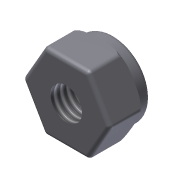
# Autodesk Inventor part: 10-32 regular lock nut
Saved by Autodesk Inventor 2013 (Build 170138000, 138)
## iProperties
Created: 2011-07-10
Part Number: 10-32 regular lock nut
Document SubType Name: Modeling
Designer: Dan Niemitalo
Density: 3.73276 g/cm^3
Material: Steel
Mass: 1.361 g
Surface Area: 3.79246 cm^2
Volume: 0.364609 cm^3
Author: Dan Niemitalo
Autodesk Inventor part; units mm, degrees
ref_plane "YZ Plane" through (0, 0, 0) normal (1, 0, 0) x (0, 1, 0)
ref_plane "XZ Plane" through (0, 0, 0) normal (0, 1, 0) x (-1, 0, 0)
ref_plane "XY Plane" through (0, 0, 0) normal (0, 0, 1) x (1, 0, 0)
sketch "Sketch1" plane through (0, 0, 0) normal (0, 0, 1) x (1, 0, 0)
  line L0 (-2.7496, 4.7625) -> (2.7496, 4.7625)
  line L1 (2.7496, 4.7625) -> (5.4993, 0)
  line L2 (5.4993, 0) -> (2.7496, -4.7625)
  line L3 (2.7496, -4.7625) -> (-2.7496, -4.7625)
  line L4 (-2.7496, -4.7625) -> (-5.4993, 0)
  line L5 (-5.4993, 0) -> (-2.7496, 4.7625)
  point P0 (0, 0)
  point P1 (0, 0)
  dimension "d0" = 9.525
  constraints: 12 end point, 1 coincident, 1 horizontal, 13 other
  measures "d0" distance between parallel lines of L3 L0
extrude "Extrusion1" add sketch "Sketch1" along normal blind 4.3656
sketch "Sketch3" plane through (0, 0, 4.3656) normal (0, 0, 1) x (1, 0, 0)
  circle A0 centre (0, 0) radius 4.572
  dimension "d3" = 9.144
  constraints: 1 centre point, 1 coincident
  measures "d3" diameter of A0
extrude "Extrusion2" add sketch "Sketch3" along normal blind 1.5875
sketch "Sketch8" plane through (0, 0, 5.9531) normal (0, 0, 1) x (1, 0, 0)
  circle A0 centre (0, 0) radius 1.9812 projected
  circle A1 centre (0, 0) radius 4.572 projected
  circle A2 centre (0, 0) radius 3.175
  dimension "d14" = 6.35
  constraints: 1 centre point, 1 coincident
  measures "d14" diameter of A2
extrude "Extrusion3" cut sketch "Sketch8" against normal blind 0.254 contours A2
sketch "Sketch9" plane through (0, 0, 0) normal (0, 0, -1) x (-1, 0, 0)
  point P0 (0, 0)
hole "Hole2" at (0, 0, 0) direction (0, 0, 1) diameter 3.9624 end through all thread size "10-32 UNF" class "2B" standard "ANSI Unified Screw Threads"
sketch "Sketch10" plane through (0, 0, 0) normal (0, 1, 0) x (-1, 0, 0)
  line L0 (-5.4993, 4.3656) -> (-2.7496, 4.3656) projected
  line L1 (-2.7496, 0) -> (-2.7496, 4.3656) projected
  line L2 (-5.4993, 0) -> (-2.7496, 0) projected
  line L3 (-5.4993, 0) -> (-5.4993, 4.3656) projected
  line L4 (0, 0) -> (0, 6.9243)
  arc A0 (-4.572, 4.3656) -> (-5.4993, 3.5232) centre (-4.572, 3.4341) ccw
  line L5 (-5.4993, 3.5232) -> (-5.4993, 4.3656)
  line L6 (-4.572, 4.3656) -> (-5.4993, 4.3656)
  dimension "d24" = 4.572
  constraints: 6 end point, 2 parallel, 2 point on circle, 2 point on line, 2 tangent, 1 centre point, 1 collinear
  measures "d24" distance from line of L4 L6.start
revolve "Revolution2" cut sketch "Sketch10" angle 360 about axis through (0, 0, 0) along (0, 0, 1) contours L0 A0 L3
fillet "Fillet1" radius 0.508 12 edges at (-2.7496, -4.7625, 1.7616) (2.7496, -4.7625, 1.7616) (5.4993, 0, 1.7616) (2.7496, 4.7625, 1.7616) (-5.4993, 0, 1.7616) (-2.7496, 4.7625, 1.7616) (0, 4.7625, 0) (4.1244, 2.3812, 0) (4.1244, -2.3813, 0) (0, -4.7625, 0) (-4.1244, -2.3812, 0) (-4.1244, 2.3813, 0)
fillet "Fillet2" radius 0.508 1 edges at (-4.572, 0, 5.9531)
body "Solid1"
